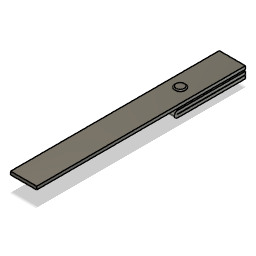
light v1 (Autodesk Fusion 360 design; units mm, degrees)
Autodesk Fusion 360 part; units mm, degrees
sketch "Esquisse1" plane through (0, 0, 0) normal (0, 1, 0) x (1, 0, 0)
  line L0 (25, 200) -> (-25, 200)
  line L1 (-25, 200) -> (-25, -200)
  line L2 (-25, -200) -> (25, -200)
  line L3 (25, -200) -> (25, 200)
  line L4 (25, 200) -> (-25, -200) construction
  line L5 (-25, 200) -> (25, -200) construction
  circle A0 centre (0, 100) radius 6.5
  circle A1 centre (0, 100) radius 4
  dimension "d1" = 50
  dimension "d2" = 400
  dimension "d3" = 13
  dimension "d4" = 8
  constraint horizontal L0
  constraint perpendicular L0 L1
  constraint parallel L0 L2
  constraint parallel L1 L3
  constraint coincident L4 origin
  constraint coincident L5 origin
  constraint concentric A0 A1
  measures "d1" distance of L1.end L2.end
  measures "d2" distance of L0.end L1.end
  measures "d3" diameter of A0
  measures "d4" diameter of A1
extrude "Extrusion1" add sketch "Esquisse1" against normal blind 6 contours L0 L1 L2 L3 makes body 1
extrude "Extrusion2" add sketch "Esquisse1" against normal blind 7 contours A0 bodies 1
fillet "Congé1" radius 3 1 edges at (-6.0601, -7, -102.3505) on bodies 1
extrude "Extrusion3" add 1 faces at (0.1619, -6, 102.1606) along direction (0, -1, 0) blind 9 and the other way blind -3 on bodies 1 bodies 1 makes body 2
extrude "Extrusion4" add sketch "Esquisse1" along normal blind -15 and the other way blind 8 contours A0 bodies 2
fillet "Congé2" radius 3 1 edges at (-6.0601, -8, -102.3505) on bodies 2
extrude "Extrusion5" add 1 faces at (0, -15, 101.3333) along direction (0, -1, 0) blind 6.5 and the other way blind -0.5 separate body on bodies 2 makes body 3
extrude "Extrusion6" add sketch "Esquisse1" along normal blind -22.5 and the other way blind 15.5 contours A0 bodies 3
fillet "Congé3" radius 3 1 edges at (-6.0601, -22.5, -102.3505) on bodies 3
extrude "Extrusion7" add sketch "Esquisse1" along normal blind 1 contours A0 bodies 1
fillet "Congé4" radius 3 1 edges at (-6.0601, 1, -97.6495) on bodies 1
extrude "Extrusion8" cut 2 faces at (-8.3333, -17.5, 200) (-8.3333, -11, 200) along direction (0, 0, -1) blind 270 on bodies 2 3 bodies 2 3
extrude "Extrusion9" add 1 faces at (-0.0996, -15, -167.9963) along direction (0, -1, 0) blind 0.25 separate body on bodies 2 makes body 4
revolve "Révolution1" add 1 faces at (-8.3333, -11, -70) angle 180 about axis through (25, -15.25, -70) along (1, 0, 0) on bodies 2 bodies 2 3 4
extrude "Extrusion10" cut 1 faces at (-0.0996, -15.25, -167.9963) along direction (0, 1, 0) blind 0.25 on bodies 2 bodies 2
sketch "Esquisse2" plane through (0, 0, 0) normal (0, -1, 0) x (1, 0, 0)
  line L0 (25, -70) -> (-25, -70)
  line L1 (-25, -70) -> (-25, -200)
  line L2 (-25, -200) -> (25, -200)
  line L3 (25, -200) -> (25, -70)
  circle A0 centre (0, -100) radius 6.5
  circle A1 centre (0, -100) radius 10
  circle A2 centre (0, -100) radius 3.5
  circle A3 centre (0, -100) radius 6.5
  line L4 (25, 200) -> (25, -200)
  line L5 (25, -200) -> (-25, -200)
  line L6 (-25, -200) -> (-25, 200)
  line L7 (-25, 200) -> (25, 200)
  dimension "d42" = 7
  constraint concentric A0 A1
  constraint concentric A1 A2
  measures "d42" diameter of A2
extrude "Extrusion11" add sketch "Esquisse2" along normal blind -1 and the other way blind 4 separate body contours A0 A3 | A1 | A2 makes body 5
fillet "Congé5" radius 2 1 edges at (-9.3233, 4, -96.3838) on bodies 5
fillet "Congé6" radius 1 1 edges at (-9.3233, 1, -96.3838) on bodies 5
extrude "Extrusion12" add sketch "Esquisse2" along normal blind 22.5 and the other way blind 1 contours A2 bodies 5
extrude "Extrusion13" add 1 faces at (1.7216, -22.5, -100.6592) along direction (0, -1, 0) blind 12 on bodies 5 bodies 5
ref_plane "Plan de construction1" through (0, 0, -100) normal (0, 0, 1) x (1, 0, 0)
sketch "Esquisse3" plane through (0, 0, -100) normal (0, 0, 1) x (1, 0, 0)
  line L0 (0, -32.5) -> (0, -22.5)
  line L1 (0, -22.5) -> (0, -22.7)
  circle A0 centre (0, -25.5) radius 1.7
  line L2 (0, -34.5) -> (-1.5, -34.5)
  line L3 (-1.5, -34.5) -> (-1.5, -32.5)
  circle A1 centre (-1.5, -32.5) radius 2
  circle A2 centre (1.5, -32.5) radius 2
  line L4 (3.5, -34.5) -> (3.5, -31.3)
  line L5 (-3.5, -34.5) -> (3.5, -34.5)
  line L6 (3.5, -34.5) -> (-3.5, -34.5)
  line L7 (-3.5, -34.5) -> (-3.5, -31.3)
  dimension "d60" = 3.4
  dimension "d65" = 1.5
  dimension "d66" = 2
  dimension "d67" = 4
  constraint vertical L0
  constraint coincident L0 L1.end
  constraint horizontal L2
  constraint perpendicular L2 L3
  constraint coincident L3.end A1.centre
  constraint symmetric L0 A1 A2
  constraint vertical L4
  constraint tangent A2 L4
  constraint coincident L4.start L5
  constraint coincident L4.start L5.end
  constraint coincident L5.start L6.end
  constraint perpendicular L6 L7
  constraint coincident L0 A0.centre
  measures "d60" diameter of A0
  measures "d65" distance of L2.start L2.end
  measures "d66" distance of L2.end L3.end
  measures "d67" diameter of A1
extrude "Extrusion14" cut sketch "Esquisse3" along normal blind 5 and the other way blind 5 contours L0 A0 | L0 A0 bodies 5
thread "Filetage2" "ISO Metric profile 7.0 M7x1 6g" major diameter 6.884 minor diameter 5.744 pitch 1 angle 60 modelled right hand crest width 0.1446 on face at (-2.0275, -19.6639, -102.8529) crest through (3.442, 1.25, -100) on bodies 5
revolve "Révolution2" cut sketch "Esquisse3" angle 360 about axis through (0, -32.5, -100) along (0, 1, 0) contours A1 L5 L6 L7 | A2 L4 L5 L6 bodies 5
sketch "Esquisse5" plane through (0, -34.5, 0) normal (0, -1, 0) x (1, 0, 0)
  circle A0 centre (0, -100) radius 1.5
  circle A1 centre (0, -100) radius 10
  circle A2 centre (0, -100) radius 3.5
  circle A3 centre (0, -100) radius 5.5
  circle A4 centre (0, -100) radius 9
  circle A5 centre (0, -100) radius 8.9
  line L0 (0, -108.9) -> (7.7076, -104.45)
  line L1 (7.7076, -104.45) -> (7.7076, -95.55)
  line L2 (7.7076, -95.55) -> (0, -91.1)
  line L3 (0, -91.1) -> (-7.7076, -95.55)
  line L4 (-7.7076, -95.55) -> (-7.7076, -104.45)
  line L5 (-7.7076, -104.45) -> (0, -108.9)
  line L6 (0, -109) -> (7.7942, -104.5)
  line L7 (7.7942, -104.5) -> (7.7942, -95.5)
  line L8 (7.7942, -95.5) -> (0, -91)
  line L9 (0, -91) -> (-7.7942, -95.5)
  line L10 (-7.7942, -95.5) -> (-7.7942, -104.5)
  line L11 (-7.7942, -104.5) -> (0, -109)
  point P0 (0, -100)
  point P1 (0, -100)
  dimension "d69" = 20
  dimension "d70" = 7
  dimension "d71" = 11
  dimension "d94" = -1
  dimension "d95" = -1.1
  constraint concentric A0 A1
  constraint concentric A1 A2
  constraint concentric A1 A3
  constraint coincident P1 P0
  constraint coincident A5 L0.start
  constraint coincident A4 L6.start
  measures "d69" diameter of A1
  measures "d70" diameter of A2
  measures "d71" diameter of A3
extrude "Extrusion16" add sketch "Esquisse5" against normal blind 7 separate body contours A2 | A3 | L0 L1 L2 L3 L4 L5 makes body 6
extrude "Extrusion19" add sketch "Esquisse5" against normal blind 7 separate body contours A1 | A4 A5 L7 | A4 A5 L8 | A4 A5 L6 | A4 A5 L9 | A5 L7 | A5 L8 | A4 A5 L11 | A5 L6 | A4 A5 L10 | A5 L9 | A5 L11 | A5 L10 makes body 7
extrude "Extrusion18" add sketch "Esquisse5" along normal blind 1 contours A0 | A1 | A2 | A3 | A4 A5 L7 | A4 A5 L8 | A5 L7 L8 | A4 A5 L6 | A5 L6 L7 | A4 A5 L9 | A5 L8 L9 | A5 L1 L7 | A5 L7 | A5 L8 | A5 L2 L8 | A5 L6 L11 | A4 A5 L11 | A5 L0 L6 | A5 L6 | A4 A5 L10 | A5 L9 L10 | A5 L9 | A5 L3 L9 | L0 L1 L2 L3 L4 L5 | A5 L10 L11 | A5 L5 L11 | A5 L11 | A5 L10 | A5 L4 L10 bodies 7
chamfer "Chanfrein1" distance 0.5 angle 45 1 edges at (-9.3233, -35.5, -103.6162) on bodies 7
thread "Filetage4" "ISO Metric profile 7.0 M7x1 6H" major diameter 7.1472 minor diameter 6.0355 pitch 1 angle 60 modelled right hand crest width 0.2748 on face at (-1.3822, -29.8333, -99.4173) crest through (3.0178, -34.25, -100) on bodies 6
sketch "Esquisse8" plane through (0, -35.5, 0) normal (0, -1, 0) x (1, 0, 0)
  circle A0 centre (0, -100) radius 9.5
  line L0 (2.1529, -103.726) -> (-0.1022, -103.7247)
  line L1 (-0.127, -102.8894) -> (4.5454, -102.9017)
  line L2 (-0.111, -93.9025) -> (0.5539, -93.9025)
  line L3 (-2.3574, -103.7233) -> (-2.561, -103.942)
  line L4 (-5.3603, -104.1349) -> (-5.7439, -103.5844)
  line L5 (0.5539, -93.9025) -> (1.0031, -94.5435)
  line L6 (2.3659, -99.2001) -> (1.1685, -97.2165)
  line L7 (1.8541, -95.7782) -> (2.2558, -96.3718)
  line L8 (1.1685, -97.2165) -> (-0.0289, -95.2329)
  line L9 (-2.561, -103.942) -> (-2.7647, -104.1607)
  line L10 (-4.7994, -102.877) -> (-0.127, -102.8894)
  line L11 (-2.4474, -98.9824) -> (-3.0749, -100.0226)
  line L12 (-3.5593, -99.1034) -> (-2.7615, -97.8938)
  line L13 (5.1426, -104.1591) -> (3.8384, -104.1591)
  line L14 (2.8468, -99.9984) -> (2.3659, -99.2001)
  line L15 (3.1814, -98.8624) -> (4.1069, -100.2645)
  line L16 (-0.1022, -103.7247) -> (-2.3574, -103.7233)
  line L17 (1.0031, -94.5435) -> (1.4523, -95.1845)
  line L18 (5.9218, -103.0086) -> (5.5322, -103.5838)
  line L19 (-4.3571, -100.3129) -> (-3.5593, -99.1034)
  line L20 (2.2558, -96.3718) -> (2.2558, -96.916)
  line L21 (-0.0521, -95.1941) -> (-0.0753, -95.1552)
  line L22 (-0.0753, -95.1552) -> (-0.117, -95.1699)
  line L23 (4.3334, -102.4614) -> (4.0822, -102.0604)
  line L24 (1.4523, -95.1845) -> (1.8541, -95.7782)
  line L25 (-2.7647, -104.1607) -> (-4.0625, -104.1478)
  line L26 (2.2558, -96.916) -> (2.2558, -97.4602)
  line L27 (-4.0625, -104.1478) -> (-5.3603, -104.1349)
  line L28 (5.0143, -101.6365) -> (5.9218, -103.0086)
  line L29 (2.2558, -97.4602) -> (3.1814, -98.8624)
  line L30 (-0.0289, -95.2329) -> (-0.0521, -95.1941)
  line L31 (3.8384, -104.1591) -> (2.5341, -104.1591)
  line L32 (-2.437, -96.8474) -> (-2.437, -96.2947)
  line L33 (4.1069, -100.2645) -> (5.0143, -101.6365)
  line L34 (3.5941, -101.2321) -> (3.3276, -100.7967)
  line L35 (-2.437, -97.4) -> (-2.437, -96.8474)
  line L36 (4.5847, -102.8623) -> (4.3334, -102.4614)
  line L37 (5.5322, -103.5838) -> (5.1426, -104.1591)
  line L38 (-3.0749, -100.0226) -> (-3.9372, -101.4498)
  line L39 (-6.1275, -103.034) -> (-6.0391, -102.8829)
  line L40 (4.0822, -102.0604) -> (3.9714, -101.864)
  line L41 (4.565, -102.882) -> (4.5847, -102.8623)
  line L42 (-0.9892, -96.5634) -> (-1.8198, -97.9422)
  line L43 (-0.117, -95.1699) -> (-0.1587, -95.1845)
  line L44 (3.3276, -100.7967) -> (2.8468, -99.9984)
  line L45 (-5.9508, -102.7319) -> (-5.1539, -101.5224)
  line L46 (-2.7615, -97.8938) -> (-2.5993, -97.6469)
  line L47 (2.5341, -104.1591) -> (2.3435, -103.9425)
  line L48 (2.3435, -103.9425) -> (2.1529, -103.726)
  line L49 (-0.7759, -93.9025) -> (-0.111, -93.9025)
  line L50 (4.5454, -102.9017) -> (4.565, -102.882)
  line L51 (-1.8198, -97.9422) -> (-2.4474, -98.9824)
  line L52 (-2.5993, -97.6469) -> (-2.437, -97.4)
  line L53 (3.9714, -101.864) -> (3.8606, -101.6675)
  line L54 (-1.6065, -95.0986) -> (-0.7759, -93.9025)
  line L55 (-0.1587, -95.1845) -> (-0.9892, -96.5634)
  line L56 (3.8606, -101.6675) -> (3.5941, -101.2321)
  line L57 (-3.9372, -101.4498) -> (-4.7994, -102.877)
  line L58 (-5.1539, -101.5224) -> (-4.3571, -100.3129)
  line L59 (-2.437, -96.2947) -> (-1.6065, -95.0986)
  line L60 (-6.0391, -102.8829) -> (-5.9508, -102.7319)
  line L61 (-5.7439, -103.5844) -> (-6.1275, -103.034)
  line L62 (0.026, -99.3269) -> (0.1067, -99.0458)
  line L63 (0.1067, -99.0458) -> (0.1873, -98.7647)
  line L64 (1.3787, -99.2969) -> (1.3509, -99.4178)
  line L65 (0.2142, -98.734) -> (0.4972, -98.6664)
  line L66 (0.2768, -100.3854) -> (-0.1004, -100.3847)
  line L67 (0.8286, -98.6012) -> (0.877, -98.6036)
  line L68 (0.2768, -100.3854) -> (-0.1004, -100.3847)
  line L69 (1.0463, -98.7229) -> (1.2157, -98.8422)
  line L70 (1.2157, -98.8422) -> (1.2972, -99.0696)
  line L71 (1.2157, -98.8422) -> (1.2972, -99.0696)
  line L72 (0.8286, -98.6012) -> (0.877, -98.6036)
  line L73 (1.3787, -99.2969) -> (1.3509, -99.4178)
  line L74 (0.2008, -98.7493) -> (0.2142, -98.734)
  line L75 (0.4658, -102.1164) -> (0.3706, -102.2306)
  line L76 (0.4972, -98.6664) -> (0.7803, -98.5988)
  line L77 (0.2739, -102.1876) -> (0.2723, -102.0304)
  line L78 (-0.358, -100.7048) -> (-0.3188, -100.9926)
  line L79 (0.2755, -102.3448) -> (0.2739, -102.1876)
  line L80 (0.2142, -98.734) -> (0.4972, -98.6664)
  line L81 (-1.3171, -100.9376) -> (-1.5364, -101.1154)
  line L82 (1.6586, -100.4178) -> (1.6881, -100.8009)
  line L83 (1.3509, -99.4178) -> (1.323, -99.5388)
  line L84 (-1.4452, -99.7767) -> (-1.5302, -99.6094)
  line L85 (1.2972, -99.0696) -> (1.3787, -99.2969)
  line L86 (1.0887, -100.9285) -> (0.893, -100.7459)
  line L87 (0.0787, -101.0119) -> (0.0787, -100.6912)
  line L88 (-0.3642, -99.0351) -> (-0.2755, -99.2969)
  line L89 (0.1067, -99.0458) -> (0.1873, -98.7647)
  line L90 (0.3706, -102.2306) -> (0.2755, -102.3448)
  line L91 (0.026, -99.3269) -> (0.1067, -99.0458)
  line L92 (-1.4452, -99.7767) -> (-1.5302, -99.6094)
  line L93 (-0.1248, -99.3119) -> (0.026, -99.3269)
  line L94 (1.2972, -99.0696) -> (1.3787, -99.2969)
  line L95 (1.3509, -99.4178) -> (1.323, -99.5388)
  line L96 (-1.7306, -101.0869) -> (-1.8219, -100.9302)
  line L97 (1.0463, -98.7229) -> (1.2157, -98.8422)
  line L98 (-0.6265, -100.6273) -> (-0.5521, -100.6281)
  line L99 (-0.4528, -98.7734) -> (-0.3642, -99.0351)
  line L100 (-0.8406, -99.9035) -> (-0.9494, -99.8781)
  line L101 (0.877, -98.6036) -> (1.0463, -98.7229)
  line L102 (-1.0851, -98.5958) -> (-0.7885, -98.665)
  line L103 (-1.4653, -98.8358) -> (-1.2752, -98.7158)
  line L104 (-0.8406, -99.9035) -> (-0.9494, -99.8781)
  line L105 (0.7803, -98.5988) -> (0.8286, -98.6012)
  line L106 (-0.492, -98.7342) -> (-0.4724, -98.7538)
  line L107 (-0.3338, -101.5494) -> (-0.3879, -101.8183)
  line L108 (-1.5662, -101.2079) -> (-1.5662, -101.3869)
  line L109 (-0.3642, -99.0351) -> (-0.2755, -99.2969)
  line L110 (0.877, -98.6036) -> (1.0463, -98.7229)
  line L111 (0.1873, -98.7647) -> (0.2008, -98.7493)
  line L112 (-0.2755, -99.2969) -> (-0.1248, -99.3119)
  line L113 (0.1873, -98.7647) -> (0.2008, -98.7493)
  line L114 (-1.5914, -99.2344) -> (-1.5675, -99.0269)
  line L115 (0.7803, -98.5988) -> (0.8286, -98.6012)
  line L116 (-0.2755, -99.2969) -> (-0.1248, -99.3119)
  line L117 (0.4972, -98.6664) -> (0.7803, -98.5988)
  line L118 (0.2008, -98.7493) -> (0.2142, -98.734)
  line L119 (0.355, -100.579) -> (0.6039, -100.8421)
  line L120 (-0.9697, -101.0386) -> (-0.7981, -100.8329)
  line L121 (-0.4724, -98.7538) -> (-0.4528, -98.7734)
  line L122 (-1.0851, -98.5958) -> (-0.7885, -98.665)
  line L123 (-0.4724, -98.7538) -> (-0.4528, -98.7734)
  line L124 (-1.6152, -99.442) -> (-1.5914, -99.2344)
  line L125 (-0.4776, -100.3839) -> (-0.5309, -100.3484)
  line L126 (-1.7218, -101.2079) -> (-1.644, -101.2079)
  line L127 (0.5142, -99.9919) -> (0.4416, -100.0846)
  line L128 (0.3252, -100.579) -> (0.3401, -100.579)
  line L129 (-1.8444, -100.0393) -> (-1.7446, -99.9463)
  line L130 (1.2845, -101.1111) -> (1.0887, -100.9285)
  line L131 (-1.052, -101.4228) -> (-1.0691, -101.2321)
  line L132 (0.369, -102.0304) -> (0.4658, -102.0304)
  line L133 (0.5867, -99.8992) -> (0.5142, -99.9919)
  line L134 (-1.6335, -101.1012) -> (-1.7306, -101.0869)
  line L135 (0.4416, -100.0846) -> (0.3592, -100.235)
  line L136 (0.893, -100.7459) -> (0.8729, -100.481)
  line L137 (0.202, -100.6351) -> (0.3252, -100.579)
  line L138 (-1.6112, -101.5199) -> (-1.6561, -101.474)
  line L139 (1.4156, -101.2065) -> (1.3378, -101.2065)
  line L140 (1.3378, -101.2065) -> (1.3378, -101.3855)
  line L141 (1.6881, -100.8009) -> (1.6079, -100.956)
  line L142 (-1.0879, -100.4842) -> (-1.0978, -100.7597)
  line L143 (0.8729, -100.481) -> (0.8528, -100.2161)
  line L144 (0.7242, -101.7216) -> (0.5957, -101.8902)
  line L145 (-1.3318, -100.031) -> (-1.0779, -100.2088)
  line L146 (-1.0582, -99.8528) -> (-1.2517, -99.8148)
  line L147 (1.6079, -100.956) -> (1.5277, -101.1111)
  line L148 (0.8528, -101.1053) -> (0.8528, -101.3292)
  line L149 (0.0787, -100.6912) -> (0.202, -100.6351)
  line L150 (-1.0978, -100.7597) -> (-1.3171, -100.9376)
  line L151 (-0.1004, -100.3847) -> (-0.4776, -100.3839)
  line L152 (1.1985, -99.7865) -> (0.8926, -99.8429)
  line L153 (-0.592, -101.9336) -> (-0.7247, -101.9336)
  line L154 (0.3592, -100.235) -> (0.2768, -100.3854)
  line L155 (1.5433, -99.9697) -> (1.629, -100.0348)
  line L156 (1.4277, -101.4725) -> (1.4606, -101.3395)
  line L157 (-0.7123, -100.1082) -> (-0.8406, -99.9035)
  line L158 (-1.0779, -100.2088) -> (-1.0879, -100.4842)
  line L159 (0.8528, -101.3292) -> (0.8528, -101.553)
  line L160 (-1.689, -101.3409) -> (-1.7218, -101.2079)
  line L161 (-1.5662, -101.5659) -> (-1.6112, -101.5199)
  line L162 (1.3378, -101.5645) -> (1.3828, -101.5185)
  line L163 (0.5142, -99.9919) -> (0.4416, -100.0846)
  line L164 (1.0942, -100.0589) -> (1.3356, -99.9016)
  line L165 (1.629, -100.0348) -> (1.6586, -100.4178)
  line L166 (-0.4534, -101.982) -> (-0.4534, -102.1513)
  line L167 (-0.5948, -102.027) -> (-0.526, -101.9835)
  line L168 (-1.6447, -99.8532) -> (-1.6152, -99.8532)
  line L169 (-0.4235, -101.8759) -> (-0.4592, -101.9336)
  line L170 (-1.9132, -100.7734) -> (-1.8788, -100.4064)
  line L171 (-0.5816, -102.1956) -> (-0.6635, -102.0705)
  line L172 (-0.4592, -101.9336) -> (-0.592, -101.9336)
  line L173 (-1.0582, -99.8528) -> (-1.2517, -99.8148)
  line L174 (0.2642, -101.861) -> (0.1715, -101.5968)
  line L175 (1.1985, -99.7865) -> (0.8926, -99.8429)
  line L176 (-0.7247, -101.9336) -> (-0.8798, -101.7736)
  line L177 (0.1715, -101.5968) -> (0.0787, -101.3326)
  line L178 (-1.6152, -99.8532) -> (-1.5858, -99.8532)
  line L179 (1.4606, -101.3395) -> (1.4934, -101.2065)
  line L180 (-0.4897, -101.9827) -> (-0.4534, -101.982)
  line L181 (0.4658, -102.0734) -> (0.4658, -102.1164)
  line L182 (-0.9494, -99.8781) -> (-1.0582, -99.8528)
  line L183 (0.5957, -101.8902) -> (0.4299, -101.8756)
  line L184 (0.2723, -102.0304) -> (0.369, -102.0304)
  line L185 (-0.3879, -101.8183) -> (-0.4235, -101.8759)
  line L186 (-0.6635, -102.0705) -> (-0.5948, -102.027)
  line L187 (1.3966, -99.9032) -> (1.4576, -99.9047)
  line L188 (-1.8219, -100.9302) -> (-1.9132, -100.7734)
  line L189 (-0.4534, -102.1513) -> (-0.4534, -102.3206)
  line L190 (-0.4765, -102.3206) -> (-0.4996, -102.3206)
  line L191 (-0.4534, -102.3206) -> (-0.4765, -102.3206)
  line L192 (-0.526, -101.9835) -> (-0.4897, -101.9827)
  line L193 (-0.4996, -102.3206) -> (-0.5816, -102.1956)
  line L194 (1.5277, -101.1111) -> (1.4061, -101.1111)
  line L195 (0.4658, -102.0304) -> (0.4658, -102.0734)
  line L196 (-1.2517, -99.8148) -> (-1.4452, -99.7767)
  line L197 (1.3378, -101.3855) -> (1.3378, -101.5645)
  line L198 (0.4416, -100.0846) -> (0.3592, -100.235)
  line L199 (-0.5309, -100.3484) -> (-0.5841, -100.3129)
  line L200 (-0.7981, -100.8329) -> (-0.6265, -100.6273)
  line L201 (0.3592, -100.235) -> (0.2768, -100.3854)
  line L202 (0.8528, -100.2161) -> (1.0942, -100.0589)
  line L203 (-1.5302, -99.6094) -> (-1.6152, -99.442)
  line L204 (-0.5841, -100.3129) -> (-0.7123, -100.1082)
  line L205 (-0.9494, -99.8781) -> (-1.0582, -99.8528)
  line L206 (-1.2752, -98.7158) -> (-1.0851, -98.5958)
  line L207 (1.4576, -99.9047) -> (1.5433, -99.9697)
  line L208 (-1.5675, -99.0269) -> (-1.5164, -98.9314)
  line L209 (1.4061, -101.1111) -> (1.2845, -101.1111)
  line L210 (-1.2517, -99.8148) -> (-1.4452, -99.7767)
  line L211 (-0.4776, -100.3839) -> (-0.5309, -100.3484)
  line L212 (-1.5164, -98.9314) -> (-1.4653, -98.8358)
  line L213 (0.5867, -99.8992) -> (0.5142, -99.9919)
  line L214 (0.8528, -101.553) -> (0.7242, -101.7216)
  line L215 (0.3401, -100.579) -> (0.355, -100.579)
  line L216 (1.2608, -99.6626) -> (1.1985, -99.7865)
  line L217 (-1.6561, -101.474) -> (-1.689, -101.3409)
  line L218 (-1.5302, -99.6094) -> (-1.6152, -99.442)
  line L219 (-1.5364, -101.1154) -> (-1.6335, -101.1012)
  line L220 (-0.3188, -100.9926) -> (-0.2797, -101.2805)
  line L221 (-1.8788, -100.4064) -> (-1.8444, -100.0393)
  line L222 (1.3828, -101.5185) -> (1.4277, -101.4725)
  line L223 (1.323, -99.5388) -> (1.2608, -99.6626)
  line L224 (-0.1004, -100.3847) -> (-0.4776, -100.3839)
  line L225 (-1.5675, -99.0269) -> (-1.5164, -98.9314)
  line L226 (-1.0691, -101.2321) -> (-1.0194, -101.1353)
  line L227 (-0.7123, -100.1082) -> (-0.8406, -99.9035)
  line L228 (-0.4528, -98.7734) -> (-0.3642, -99.0351)
  line L229 (-1.5914, -99.2344) -> (-1.5675, -99.0269)
  line L230 (-0.1248, -99.3119) -> (0.026, -99.3269)
  line L231 (0.6039, -100.8421) -> (0.8528, -101.1053)
  line L232 (1.323, -99.5388) -> (1.2608, -99.6626)
  line L233 (-1.5662, -101.3869) -> (-1.5662, -101.5659)
  line L234 (-1.4653, -98.8358) -> (-1.2752, -98.7158)
  line L235 (-1.644, -101.2079) -> (-1.5662, -101.2079)
  line L236 (-0.4178, -100.6668) -> (-0.358, -100.7048)
  line L237 (-0.7885, -98.665) -> (-0.492, -98.7342)
  line L238 (-1.5164, -98.9314) -> (-1.4653, -98.8358)
  line L239 (0.0787, -101.3326) -> (0.0787, -101.0119)
  line L240 (-0.492, -98.7342) -> (-0.4724, -98.7538)
  line L241 (-1.7446, -99.9463) -> (-1.6447, -99.8532)
  line L242 (1.2608, -99.6626) -> (1.1985, -99.7865)
  line L243 (-0.7885, -98.665) -> (-0.492, -98.7342)
  line L244 (-0.5521, -100.6281) -> (-0.4776, -100.6288)
  line L245 (-0.4776, -100.6288) -> (-0.4178, -100.6668)
  line L246 (1.3356, -99.9016) -> (1.3966, -99.9032)
  line L247 (-1.0349, -101.6136) -> (-1.052, -101.4228)
  line L248 (0.8926, -99.8429) -> (0.5867, -99.8992)
  line L249 (-0.5841, -100.3129) -> (-0.7123, -100.1082)
  line L250 (-0.2797, -101.2805) -> (-0.3338, -101.5494)
  line L251 (0.4299, -101.8756) -> (0.2642, -101.861)
  line L252 (-1.0194, -101.1353) -> (-0.9697, -101.0386)
  line L253 (1.4934, -101.2065) -> (1.4156, -101.2065)
  line L254 (-0.5309, -100.3484) -> (-0.5841, -100.3129)
  line L255 (-1.6152, -99.442) -> (-1.5914, -99.2344)
  line L256 (-1.5858, -99.8532) -> (-1.3318, -100.031)
  line L257 (-0.8798, -101.7736) -> (-1.0349, -101.6136)
  line L258 (0.8926, -99.8429) -> (0.5867, -99.8992)
  line L259 (-1.2752, -98.7158) -> (-1.0851, -98.5958)
  dimension "d114" = 0
emboss "Gravure en relief2" depth -0.4 profiles "Esquisse8" section 1 contours L0 L2 L3 L4 L5 L7 L9 L12 L13 L15 L16 L17 L18 L19 L20 L24 L25 L26 L27 L28 L29 L31 L32 L33 L35 L37 L39 L45 L46 L47 L48 L49 L52 L54 L58 L59 L60 L61 | L62 L63 L64 L65 L66 L67 L68 L69 L70 L71 L72 L73 L74 L76 L80 L83 L84 L85 L88 L89 L91 L92 L93 L94 L95 L97 L99 L100 L101 L102 L103 L104 L105 L106 L109 L110 L111 L112 L113 L114 L115 L116 L117 L118 L121 L122 L123 L124 L125 L127 L133 L135 L146 L151 L152 L154 L157 L163 L173 L175 L182 L196 L198 L199 L201 L203 L204 L205 L206 L208 L210 L211 L212 L213 L216 L218 L223 L224 L225 L227 L228 L229 L230 L232 L234 L237 L238 L240 L242 L243 L248 L249 L254 L255 L258 L259 | L75 L77 L79 L90 L132 L181 L184 L195 | L78 L98 L107 L120 L131 L153 L169 L172 L176 L185 L200 L220 L226 L236 L244 L245 L247 L250 L252 L257 | L81 L96 L129 L134 L142 L145 L150 L158 L168 L170 L178 L188 L219 L221 L241 L256 | L82 L86 L130 L136 L141 L143 L147 L155 L164 L165 L187 L194 L202 L207 L209 L246 | L87 L119 L128 L137 L144 L148 L149 L159 L174 L177 L183 L214 L215 L231 L239 L251 | L108 L126 L138 L160 L161 L217 L233 L235 | L139 L140 L156 L162 L179 L197 L222 L253 | L166 L167 L171 L180 L186 L189 L190 L191 L192 L193 onto face at (-0.0584, -35.5, -92.9045) on bodies 7 bodies 7
sketch "Esquisse9" plane through (0, 0, 0) normal (0, 0, 1) x (1, 0, 0)
  spline S0 degree 3 poles (5.4127, -28.6266) (5.517, -28.731) (5.5206, -28.7549) (5.5192, -29.3414) knots 0 0 0 0 1 1 1 1
  spline S1 degree 3 poles (5.5192, -29.3414) (5.5173, -30.1912) (5.5184, -30.1902) (4.5558, -30.1902) knots 0 0 0 0 1 1 1 1
  line L0 (4.5558, -30.1902) -> (3.8931, -30.1902)
  line L1 (3.8931, -30.1902) -> (3.8931, -30.0142)
  line L2 (3.8931, -30.0142) -> (3.8931, -29.8383)
  line L3 (3.8931, -29.8383) -> (4.5309, -29.8383)
  line L4 (4.5309, -29.8383) -> (5.1687, -29.8383)
  line L5 (5.1687, -29.8383) -> (5.1687, -29.3544)
  line L6 (5.1687, -29.3544) -> (5.1687, -28.8705)
  line L7 (5.1687, -28.8705) -> (4.5309, -28.8705)
  line L8 (4.5309, -28.8705) -> (3.8931, -28.8705)
  line L9 (3.8931, -28.8705) -> (3.8931, -28.6946)
  line L10 (3.8931, -28.6946) -> (3.8931, -28.5186)
  line L11 (3.8931, -28.5186) -> (4.5989, -28.5186)
  spline S2 degree 3 poles (4.5989, -28.5186) (5.2896, -28.5186) (5.307, -28.521) (5.4127, -28.6266) knots 0 0 0 0 1 1 1 1
  spline S3 degree 3 poles (3.4312, -28.5712) (3.4796, -28.5986) (3.5337, -28.6426) (3.5515, -28.6688) knots 0 0 0 0 1 1 1 1
  spline S4 degree 3 poles (3.5515, -28.6688) (3.5693, -28.6951) (3.5841, -29.0055) (3.5845, -29.3586) knots 0 0 0 0 1 1 1 1
  spline S5 degree 3 poles (3.5845, -29.3586) (3.5853, -30.1868) (3.6064, -30.1624) (2.8729, -30.183) knots 0 0 0 0 1 1 1 1
  spline S6 degree 3 poles (2.8729, -30.183) (2.283, -30.1995) (2.1696, -30.1823) (2.0445, -30.0571) knots 0 0 0 0 1 1 1 1
  spline S7 degree 3 poles (2.0445, -30.0571) (1.9662, -29.9789) (1.9576, -29.9089) (1.9576, -29.3524) knots 0 0 0 0 1 1 1 1
  spline S8 degree 3 poles (1.9576, -29.3524) (1.9576, -28.7551) (1.9612, -28.731) (2.0656, -28.6266) knots 0 0 0 0 1 1 1 1
  spline S9 degree 3 poles (2.0656, -28.6266) (2.1695, -28.5226) (2.1952, -28.5187) (2.7584, -28.52) knots 0 0 0 0 1 1 1 1
  spline S10 degree 3 poles (2.7584, -28.52) (3.1108, -28.5208) (3.3782, -28.5411) (3.4312, -28.5712) knots 0 0 0 0 1 1 1 1
  line L12 (2.3095, -29.3544) -> (2.3095, -29.8383)
  line L13 (2.3095, -29.8383) -> (2.7934, -29.8383)
  line L14 (2.7934, -29.8383) -> (3.2772, -29.8383)
  line L15 (3.2772, -29.8383) -> (3.2772, -29.3544)
  line L16 (3.2772, -29.3544) -> (3.2772, -28.8705)
  line L17 (3.2772, -28.8705) -> (2.7934, -28.8705)
  line L18 (2.7934, -28.8705) -> (2.3095, -28.8705)
  line L19 (2.3095, -28.8705) -> (2.3095, -29.3544)
  line L20 (1.6497, -29.3544) -> (1.6497, -30.1902)
  line L21 (1.6497, -30.1902) -> (1.5047, -30.1902)
  spline S11 degree 3 poles (1.5047, -30.1902) (1.3408, -30.1902) (1.2589, -30.1146) (0.7219, -29.4677) knots 0 0 0 0 1 1 1 1
  line L22 (0.7219, -29.4677) -> (0.396, -29.0751)
  line L23 (0.396, -29.0751) -> (0.374, -29.6217)
  line L24 (0.374, -29.6217) -> (0.352, -30.1682)
  line L25 (0.352, -30.1682) -> (0.1871, -30.1818)
  line L26 (0.1871, -30.1818) -> (0.0221, -30.1955)
  line L27 (0.0221, -30.1955) -> (0.0221, -29.3571)
  line L28 (0.0221, -29.3571) -> (0.0221, -28.5186)
  line L29 (0.0221, -28.5186) -> (0.1947, -28.5186)
  spline S12 degree 3 poles (0.1947, -28.5186) (0.3614, -28.5186) (0.3832, -28.5374) (0.8435, -29.0786) knots 0 0 0 0 1 1 1 1
  line L30 (0.8435, -29.0786) -> (1.3198, -29.6385)
  line L31 (1.3198, -29.6385) -> (1.3321, -29.0786)
  line L32 (1.3321, -29.0786) -> (1.3444, -28.5186)
  line L33 (1.3444, -28.5186) -> (1.497, -28.5186)
  line L34 (1.497, -28.5186) -> (1.6497, -28.5186)
  line L35 (1.6497, -28.5186) -> (1.6497, -29.3544)
  spline S13 degree 3 poles (-0.4017, -28.6098) (-0.2858, -28.701) (-0.2858, -28.7012) (-0.2858, -29.3508) knots 0 0 0 0 1 1 1 1
  spline S14 degree 3 poles (-0.2858, -29.3508) (-0.2858, -30.2109) (-0.2343, -30.1636) (-1.192, -30.1821) knots 0 0 0 0 1 1 1 1
  line L36 (-1.192, -30.1821) -> (-1.9133, -30.1961)
  line L37 (-1.9133, -30.1961) -> (-1.9133, -30.0172)
  line L38 (-1.9133, -30.0172) -> (-1.9133, -29.8383)
  line L39 (-1.9133, -29.8383) -> (-1.2535, -29.8383)
  line L40 (-1.2535, -29.8383) -> (-0.5937, -29.8383)
  line L41 (-0.5937, -29.8383) -> (-0.5937, -29.3544)
  line L42 (-0.5937, -29.3544) -> (-0.5937, -28.8705)
  line L43 (-0.5937, -28.8705) -> (-1.2535, -28.8705)
  line L44 (-1.2535, -28.8705) -> (-1.9133, -28.8705)
  line L45 (-1.9133, -28.8705) -> (-1.9133, -28.6946)
  line L46 (-1.9133, -28.6946) -> (-1.9133, -28.5186)
  line L47 (-1.9133, -28.5186) -> (-1.2155, -28.5186)
  spline S15 degree 3 poles (-1.2155, -28.5186) (-0.576, -28.5186) (-0.5079, -28.5263) (-0.4017, -28.6098) knots 0 0 0 0 1 1 1 1
  line L48 (-3.101, -29.1785) -> (-3.101, -29.8383)
  line L49 (-3.101, -29.8383) -> (-2.5732, -29.8383)
  line L50 (-2.5732, -29.8383) -> (-2.0453, -29.8383)
  line L51 (-2.0453, -29.8383) -> (-2.0453, -30.0142)
  line L52 (-2.0453, -30.0142) -> (-2.0453, -30.1902)
  line L53 (-2.0453, -30.1902) -> (-2.6112, -30.1902)
  spline S16 degree 3 poles (-2.6112, -30.1902) (-3.1171, -30.1902) (-3.1894, -30.1805) (-3.293, -30.099) knots 0 0 0 0 1 1 1 1
  line L54 (-3.293, -30.099) -> (-3.4089, -30.0078)
  line L55 (-3.4089, -30.0078) -> (-3.4089, -29.2632)
  line L56 (-3.4089, -29.2632) -> (-3.4089, -28.5186)
  line L57 (-3.4089, -28.5186) -> (-3.255, -28.5186)
  line L58 (-3.255, -28.5186) -> (-3.101, -28.5186)
  line L59 (-3.101, -28.5186) -> (-3.101, -29.1785)
  line L60 (-3.7269, -29.3434) -> (-3.7388, -30.1682)
  line L61 (-3.7388, -30.1682) -> (-4.4575, -30.1682)
  line L62 (-4.4575, -30.1682) -> (-5.1762, -30.1682)
  line L63 (-5.1762, -30.1682) -> (-5.2823, -30.0448)
  spline S17 degree 3 poles (-5.2823, -30.0448) (-5.4275, -29.8758) (-5.4369, -29.3839) (-5.2982, -29.2077) knots 0 0 0 0 1 1 1 1
  spline S18 degree 3 poles (-5.2982, -29.2077) (-5.2106, -29.0963) (-5.1923, -29.0927) (-4.6494, -29.0808) knots 0 0 0 0 1 1 1 1
  line L64 (-4.6494, -29.0808) -> (-4.0907, -29.0685)
  line L65 (-4.0907, -29.0685) -> (-4.0776, -28.7936)
  line L66 (-4.0776, -28.7936) -> (-4.0646, -28.5186)
  line L67 (-4.0646, -28.5186) -> (-3.8897, -28.5186)
  line L68 (-3.8897, -28.5186) -> (-3.7149, -28.5186)
  line L69 (-3.7149, -28.5186) -> (-3.7269, -29.3434)
  line L70 (-5.0279, -29.6293) -> (-5.0413, -29.8383)
  line L71 (-5.0413, -29.8383) -> (-4.555, -29.8383)
  line L72 (-4.555, -29.8383) -> (-4.0687, -29.8383)
  line L73 (-4.0687, -29.8383) -> (-4.0687, -29.6169)
  line L74 (-4.0687, -29.6169) -> (-4.0687, -29.3954)
  line L75 (-4.0687, -29.3954) -> (-4.5416, -29.4079)
  line L76 (-4.5416, -29.4079) -> (-5.0145, -29.4204)
  line L77 (-5.0145, -29.4204) -> (-5.0279, -29.6293)
  line L78 (5.6526, -32.3218) -> (5.6526, -34.0171)
  line L79 (5.6526, -34.0171) -> (4.1855, -34.0171)
  spline S19 degree 3 poles (4.1855, -34.0171) (2.7365, -34.0171) (2.7166, -34.0159) (2.573, -33.9181) knots 0 0 0 0 1 1 1 1
  spline S20 degree 3 poles (2.573, -33.9181) (2.2786, -33.7178) (2.2451, -33.6298) (2.2283, -33.0115) knots 0 0 0 0 1 1 1 1
  spline S21 degree 3 poles (2.2283, -33.0115) (2.2196, -32.6895) (2.2338, -32.3754) (2.2618, -32.2716) knots 0 0 0 0 1 1 1 1
  spline S22 degree 3 poles (2.2618, -32.2716) (2.3233, -32.0432) (2.6071, -31.7737) (2.7862, -31.7737) knots 0 0 0 0 1 1 1 1
  spline S23 degree 3 poles (2.7862, -31.7737) (2.8546, -31.7737) (2.9225, -31.7619) (2.9369, -31.7475) knots 0 0 0 0 1 1 1 1
  spline S24 degree 3 poles (2.9369, -31.7475) (2.9514, -31.733) (2.7963, -31.5243) (2.5924, -31.2837) knots 0 0 0 0 1 1 1 1
  spline S25 degree 3 poles (2.5924, -31.2837) (2.3465, -30.9937) (2.2215, -30.8099) (2.2215, -30.7382) knots 0 0 0 0 1 1 1 1
  spline S26 degree 3 poles (2.2215, -30.7382) (2.2215, -30.6315) (2.2268, -30.63) (2.6082, -30.63) knots 0 0 0 0 1 1 1 1
  line L80 (2.6082, -30.63) -> (2.995, -30.63)
  line L81 (2.995, -30.63) -> (3.4668, -31.2019)
  line L82 (3.4668, -31.2019) -> (3.9387, -31.7737)
  line L83 (3.9387, -31.7737) -> (4.4011, -31.7737)
  spline S27 degree 3 poles (4.4011, -31.7737) (4.7617, -31.7737) (4.8689, -31.7599) (4.8877, -31.7108) knots 0 0 0 0 1 1 1 1
  spline S28 degree 3 poles (4.8877, -31.7108) (4.901, -31.6762) (4.9152, -31.4238) (4.9193, -31.1499) knots 0 0 0 0 1 1 1 1
  line L84 (4.9193, -31.1499) -> (4.9268, -30.652)
  line L85 (4.9268, -30.652) -> (5.2897, -30.6393)
  line L86 (5.2897, -30.6393) -> (5.6526, -30.6265)
  line L87 (5.6526, -30.6265) -> (5.6526, -32.3218)
  line L88 (2.9693, -32.8954) -> (2.9693, -33.3133)
  line L89 (2.9693, -33.3133) -> (3.9371, -33.3133)
  spline S29 degree 3 poles (3.9371, -33.3133) (4.5511, -33.3133) (4.9058, -33.2972) (4.9075, -33.2693) knots 0 0 0 0 1 1 1 1
  spline S30 degree 3 poles (4.9075, -33.2693) (4.9091, -33.2451) (4.9103, -33.1165) (4.9103, -32.9834) knots 0 0 0 0 1 1 1 1
  spline S31 degree 3 poles (4.9103, -32.9834) (4.9103, -32.8503) (4.9091, -32.6821) (4.9075, -32.6095) knots 0 0 0 0 1 1 1 1
  line L90 (4.9075, -32.6095) -> (4.9048, -32.4775)
  line L91 (4.9048, -32.4775) -> (3.9371, -32.4775)
  line L92 (3.9371, -32.4775) -> (2.9693, -32.4775)
  line L93 (2.9693, -32.4775) -> (2.9693, -32.8954)
  spline S32 degree 3 poles (1.3409, -30.7071) (1.4251, -30.7494) (1.5389, -30.8513) (1.5938, -30.9335) knots 0 0 0 0 1 1 1 1
  spline S33 degree 3 poles (1.5938, -30.9335) (1.6926, -31.0814) (1.6937, -31.098) (1.6937, -32.55) knots 0 0 0 0 1 1 1 1
  line L94 (1.6937, -32.55) -> (1.6937, -34.0171)
  line L95 (1.6937, -34.0171) -> (1.3418, -34.0171)
  line L96 (1.3418, -34.0171) -> (0.9899, -34.0171)
  line L97 (0.9899, -34.0171) -> (0.9899, -32.6746)
  line L98 (0.9899, -32.6746) -> (0.9899, -31.3322)
  line L99 (0.9899, -31.3322) -> (0.0111, -31.344)
  line L100 (0.0111, -31.344) -> (-0.9676, -31.3558)
  line L101 (-0.9676, -31.3558) -> (-0.9792, -32.6865)
  line L102 (-0.9792, -32.6865) -> (-0.9909, -34.0171)
  line L103 (-0.9909, -34.0171) -> (-1.3438, -34.0171)
  line L104 (-1.3438, -34.0171) -> (-1.6968, -34.0171)
  line L105 (-1.6968, -34.0171) -> (-1.6841, -32.5467)
  spline S34 degree 3 poles (-1.6841, -32.5467) (-1.6719, -31.134) (-1.6678, -31.0714) (-1.5794, -30.9521) knots 0 0 0 0 1 1 1 1
  spline S35 degree 3 poles (-1.5794, -30.9521) (-1.5288, -30.8838) (-1.4219, -30.7835) (-1.3419, -30.729) knots 0 0 0 0 1 1 1 1
  spline S36 degree 3 poles (-1.3419, -30.729) (-1.2, -30.6324) (-1.1683, -30.63) (-0.0044, -30.6301) knots 0 0 0 0 1 1 1 1
  spline S37 degree 3 poles (-0.0044, -30.6301) (1.0429, -30.6302) (1.2064, -30.6395) (1.3409, -30.7071) knots 0 0 0 0 1 1 1 1
  spline S38 degree 3 poles (-2.5727, -30.729) (-2.35, -30.8806) (-2.2632, -31.0281) (-2.2348, -31.3034) knots 0 0 0 0 1 1 1 1
  line L106 (-2.2348, -31.3034) -> (-2.2089, -31.5538)
  line L107 (-2.2089, -31.5538) -> (-2.567, -31.5538)
  spline S39 degree 3 poles (-2.567, -31.5538) (-2.9196, -31.5538) (-2.9251, -31.5521) (-2.9251, -31.4438) knots 0 0 0 0 1 1 1 1
  line L108 (-2.9251, -31.4438) -> (-2.9251, -31.3339)
  line L109 (-2.9251, -31.3339) -> (-3.8928, -31.3339)
  line L110 (-3.8928, -31.3339) -> (-4.8605, -31.3339)
  line L111 (-4.8605, -31.3339) -> (-4.8605, -31.6638)
  line L112 (-4.8605, -31.6638) -> (-4.8605, -31.9937)
  line L113 (-4.8605, -31.9937) -> (-3.8268, -31.9937)
  line L114 (-3.8268, -31.9937) -> (-2.7931, -31.9937)
  line L115 (-2.7931, -31.9937) -> (-2.7931, -32.3456)
  line L116 (-2.7931, -32.3456) -> (-2.7931, -32.6975)
  line L117 (-2.7931, -32.6975) -> (-3.7608, -32.6975)
  line L118 (-3.7608, -32.6975) -> (-4.7286, -32.6975)
  line L119 (-4.7286, -32.6975) -> (-4.7286, -33.0054)
  line L120 (-4.7286, -33.0054) -> (-4.7286, -33.3133)
  line L121 (-4.7286, -33.3133) -> (-3.8268, -33.3133)
  line L122 (-3.8268, -33.3133) -> (-2.9251, -33.3133)
  line L123 (-2.9251, -33.3133) -> (-2.9251, -33.1813)
  line L124 (-2.9251, -33.1813) -> (-2.9251, -33.0494)
  line L125 (-2.9251, -33.0494) -> (-2.5732, -33.0494)
  line L126 (-2.5732, -33.0494) -> (-2.2213, -33.0494)
  line L127 (-2.2213, -33.0494) -> (-2.2215, -33.2143)
  spline S40 degree 3 poles (-2.2215, -33.2143) (-2.222, -33.4836) (-2.2987, -33.6817) (-2.4652, -33.8431) knots 0 0 0 0 1 1 1 1
  line L128 (-2.4652, -33.8431) -> (-2.6219, -33.9951)
  line L129 (-2.6219, -33.9951) -> (-3.7962, -34.0071)
  spline S41 degree 3 poles (-3.7962, -34.0071) (-4.9077, -34.0184) (-4.9782, -34.0143) (-5.1139, -33.9305) knots 0 0 0 0 1 1 1 1
  spline S42 degree 3 poles (-5.1139, -33.9305) (-5.384, -33.7637) (-5.4321, -33.6234) (-5.4323, -33.0012) knots 0 0 0 0 1 1 1 1
  spline S43 degree 3 poles (-5.4323, -33.0012) (-5.4324, -32.5846) (-5.4497, -32.4125) (-5.5019, -32.3078) knots 0 0 0 0 1 1 1 1
  spline S44 degree 3 poles (-5.5019, -32.3078) (-5.5571, -32.1972) (-5.5684, -32.0517) (-5.5569, -31.6003) knots 0 0 0 0 1 1 1 1
  spline S45 degree 3 poles (-5.5569, -31.6003) (-5.5443, -31.1087) (-5.5301, -31.0153) (-5.4513, -30.908) knots 0 0 0 0 1 1 1 1
  spline S46 degree 3 poles (-5.4513, -30.908) (-5.258, -30.6449) (-5.1753, -30.6302) (-3.8884, -30.6301) knots 0 0 0 0 1 1 1 1
  spline S47 degree 3 poles (-3.8884, -30.6301) (-2.7472, -30.63) (-2.7146, -30.6325) (-2.5728, -30.729) knots 0 0 0 0 1 1 1 1
  line L130 (-2.5728, -30.729) -> (-2.5727, -30.729)
  line L131 (12.4282, -29.8931) -> (12.3373, -30.0741)
  line L132 (11.7412, -30.8828) -> (12.0939, -30.653)
  line L133 (8.9096, -28.5153) -> (9.3429, -28.6164)
  line L134 (12.5357, -30.4255) -> (12.6248, -30.4278)
  line L135 (12.4466, -30.4233) -> (12.5357, -30.4255)
  line L136 (10.533, -29.5835) -> (10.6509, -29.1727)
  line L137 (9.8048, -28.7461) -> (9.8334, -28.7747)
  line L138 (12.0939, -30.653) -> (12.4466, -30.4233)
  line L139 (9.3429, -28.6164) -> (9.7762, -28.7175)
  line L140 (11.1403, -30.6906) -> (11.0199, -30.9104)
  line L141 (12.7501, -30.5228) -> (12.8753, -30.6179)
  line L142 (9.5797, -31.4837) -> (9.6884, -31.4848)
  line L143 (11.2216, -28.6184) -> (11.6351, -28.5196)
  line L144 (11.7993, -30.3374) -> (11.3524, -30.4198)
  line L145 (12.3905, -29.2075) -> (12.5095, -29.5396)
  line L146 (8.354, -28.866) -> (8.6318, -28.6907)
  line L147 (9.2669, -30.426) -> (9.1079, -30.389)
  line L148 (9.1079, -30.389) -> (8.9489, -30.352)
  line L149 (8.1698, -29.4484) -> (8.2047, -29.1451)
  line L150 (9.7972, -31.128) -> (9.7194, -31.0761)
  line L151 (12.6248, -30.4278) -> (12.7501, -30.5228)
  line L152 (10.7688, -28.762) -> (10.7884, -28.7396)
  line L153 (10.0925, -29.5396) -> (10.3128, -29.5616)
  line L154 (8.6318, -28.6907) -> (8.9096, -28.5153)
  line L155 (11.3524, -30.4198) -> (11.2463, -30.5552)
  line L156 (12.3373, -30.0741) -> (12.2463, -30.255)
  line L157 (9.7194, -31.0761) -> (9.6416, -31.0242)
  line L158 (11.0138, -31.413) -> (11.3775, -31.7975)
  line L159 (12.5095, -29.5396) -> (12.4689, -29.7164)
  line L160 (7.946, -30.4885) -> (8.0919, -30.3526)
  line L161 (11.1769, -33.658) -> (11.0366, -33.8263)
  line L162 (9.8846, -31.5414) -> (9.972, -31.5969)
  line L163 (11.1233, -33.3076) -> (10.8811, -33.2863)
  line L164 (8.9489, -30.352) -> (8.6661, -30.2964)
  line L165 (10.9702, -31.413) -> (10.992, -31.413)
  line L166 (10.8929, -33.5337) -> (11.0342, -33.5337)
  line L167 (10.3128, -29.5616) -> (10.533, -29.5835)
  line L168 (11.6351, -28.5196) -> (11.7058, -28.5232)
  line L169 (12.0239, -28.701) -> (12.2714, -28.8754)
  line L170 (10.8811, -33.2863) -> (10.7456, -32.9002)
  line L171 (8.178, -30.3526) -> (8.549, -30.6123)
  line L172 (11.3654, -33.3289) -> (11.1233, -33.3076)
  line L173 (10.8994, -31.1302) -> (10.3483, -31.1291)
  line L174 (8.3833, -30.2408) -> (8.2591, -29.9963)
  line L175 (10.8081, -28.7172) -> (11.2216, -28.6184)
  line L176 (11.7765, -28.5267) -> (12.0239, -28.701)
  line L177 (9.4542, -30.7251) -> (9.2669, -30.426)
  line L178 (10.8976, -33.9932) -> (10.8952, -33.7635)
  line L179 (8.2591, -29.9963) -> (8.1349, -29.7517)
  line L180 (8.2047, -29.1451) -> (8.2794, -29.0056)
  line L181 (8.549, -30.6123) -> (8.92, -30.8721)
  line L182 (10.7884, -28.7396) -> (10.8081, -28.7172)
  line L183 (8.1349, -30.3526) -> (8.178, -30.3526)
  line L184 (12.2463, -30.255) -> (11.7993, -30.3374)
  line L185 (9.7762, -28.7175) -> (9.8048, -28.7461)
  line L186 (11.0366, -33.8263) -> (10.8976, -33.9932)
  line L187 (11.1756, -33.5966) -> (11.1769, -33.658)
  line L188 (8.1349, -29.7517) -> (8.1698, -29.4484)
  line L189 (8.6661, -30.2964) -> (8.3833, -30.2408)
  line L190 (12.4689, -29.7164) -> (12.4282, -29.8931)
  line L191 (10.6101, -32.5141) -> (10.6101, -32.0456)
  line L192 (11.2463, -30.5552) -> (11.1403, -30.6906)
  line L193 (11.7058, -28.5232) -> (11.7765, -28.5267)
  line L194 (8.0919, -30.3526) -> (8.1349, -30.3526)
  line L195 (12.8753, -30.6179) -> (12.9185, -31.1776)
  line L196 (9.6301, -33.3923) -> (9.4361, -33.3923)
  line L197 (10.6101, -32.0456) -> (10.6101, -31.5771)
  line L198 (7.7498, -31.1608) -> (7.8001, -30.6244)
  line L199 (12.3719, -32.1906) -> (12.0859, -31.9238)
  line L200 (9.8242, -33.3923) -> (9.6301, -33.3923)
  line L201 (9.6416, -31.0242) -> (9.4542, -30.7251)
  line L202 (7.9663, -32.1552) -> (7.8329, -31.9262)
  line L203 (9.7651, -33.9579) -> (9.6453, -33.7751)
  line L204 (9.5256, -33.5924) -> (9.626, -33.5288)
  line L205 (10.0864, -32.438) -> (10.0073, -32.8309)
  line L206 (8.9829, -32.9248) -> (8.9579, -32.646)
  line L207 (9.2095, -33.1586) -> (8.9829, -32.9248)
  line L208 (9.0782, -32.0845) -> (9.3289, -31.7841)
  line L209 (11.7705, -31.2699) -> (11.7412, -30.8828)
  line L210 (11.3775, -31.7975) -> (11.7412, -32.1821)
  line L211 (8.2501, -32.1968) -> (8.1082, -32.176)
  line L212 (8.2066, -32.8551) -> (8.1409, -32.7879)
  line L213 (8.0929, -32.332) -> (8.2066, -32.332)
  line L214 (11.0199, -30.9104) -> (10.8994, -31.1302)
  line L215 (9.626, -33.5288) -> (9.7265, -33.4652)
  line L216 (8.92, -30.8721) -> (8.9055, -31.2746)
  line L217 (8.1409, -32.7879) -> (8.0752, -32.7208)
  line L218 (7.9792, -32.332) -> (8.0929, -32.332)
  line L219 (8.0752, -32.7208) -> (8.0272, -32.5264)
  line L220 (8.1082, -32.176) -> (7.9663, -32.1552)
  line L221 (9.972, -31.5969) -> (10.0292, -32.0174)
  line L222 (9.6453, -33.7751) -> (9.5256, -33.5924)
  line L223 (8.0272, -32.5264) -> (7.9792, -32.332)
  line L224 (12.9616, -31.7373) -> (12.8444, -31.9639)
  line L225 (8.5705, -31.937) -> (8.2501, -32.1968)
  line L226 (12.5496, -32.1906) -> (12.3719, -32.1906)
  line L227 (10.8952, -33.7635) -> (10.8929, -33.5337)
  line L228 (10.6509, -29.1727) -> (10.7688, -28.762)
  line L229 (12.4498, -32.3299) -> (12.4498, -32.5914)
  line L230 (12.9185, -31.1776) -> (12.9616, -31.7373)
  line L231 (11.0342, -33.5337) -> (11.1756, -33.5337)
  line L232 (9.8334, -28.7747) -> (9.963, -29.1572)
  line L233 (8.9055, -31.2746) -> (8.891, -31.6771)
  line L234 (8.9329, -32.3673) -> (9.0055, -32.2259)
  line L235 (12.4498, -32.5914) -> (12.4498, -32.853)
  line L236 (12.5812, -32.7187) -> (12.6292, -32.5243)
  line L237 (7.8329, -31.9262) -> (7.6996, -31.6971)
  line L238 (9.0055, -32.2259) -> (9.0782, -32.0845)
  line L239 (9.963, -29.1572) -> (10.0925, -29.5396)
  line L240 (10.3483, -31.1291) -> (9.7972, -31.128)
  line L241 (8.2066, -32.5935) -> (8.2066, -32.8551)
  line L242 (9.8325, -33.463) -> (9.8325, -33.7105)
  line L243 (8.891, -31.6771) -> (8.5705, -31.937)
  line L244 (10.7902, -31.495) -> (10.9702, -31.413)
  line L245 (11.7412, -32.8362) -> (11.5533, -33.0825)
  line L246 (11.5533, -33.0825) -> (11.3654, -33.3289)
  line L247 (12.8444, -31.9639) -> (12.7272, -32.1906)
  line L248 (12.6292, -32.5243) -> (12.6772, -32.3299)
  line L249 (10.992, -31.413) -> (11.0138, -31.413)
  line L250 (9.7988, -33.9579) -> (9.7651, -33.9579)
  line L251 (9.4361, -33.3923) -> (9.2095, -33.1586)
  line L252 (8.2794, -29.0056) -> (8.354, -28.866)
  line L253 (9.7795, -33.4641) -> (9.8325, -33.463)
  line L254 (7.6996, -31.6971) -> (7.7498, -31.1608)
  line L255 (12.6772, -32.3299) -> (12.5635, -32.3299)
  line L256 (12.2714, -28.8754) -> (12.3905, -29.2075)
  line L257 (11.7412, -32.5092) -> (11.7412, -32.8362)
  line L258 (12.7272, -32.1906) -> (12.5496, -32.1906)
  line L259 (12.0859, -31.9238) -> (11.7999, -31.657)
  line L260 (9.7972, -31.4858) -> (9.8846, -31.5414)
  line L261 (10.7456, -32.9002) -> (10.6101, -32.5141)
  line L262 (7.8001, -30.6244) -> (7.946, -30.4885)
  line L263 (9.8762, -33.3081) -> (9.8242, -33.3923)
  line L264 (9.8325, -33.9579) -> (9.7988, -33.9579)
  line L265 (10.0292, -32.0174) -> (10.0864, -32.438)
  line L266 (9.6884, -31.4848) -> (9.7972, -31.4858)
  line L267 (11.1756, -33.5337) -> (11.1756, -33.5966)
  line L268 (9.3289, -31.7841) -> (9.5797, -31.4837)
  line L269 (11.7412, -32.1821) -> (11.7412, -32.5092)
  line L270 (12.4498, -32.853) -> (12.5155, -32.7858)
  line L271 (8.9579, -32.646) -> (8.9329, -32.3673)
  line L272 (12.5635, -32.3299) -> (12.4498, -32.3299)
  line L273 (9.7265, -33.4652) -> (9.7795, -33.4641)
  line L274 (8.2066, -32.332) -> (8.2066, -32.5935)
  line L275 (9.8325, -33.7105) -> (9.8325, -33.9579)
  line L276 (10.6101, -31.5771) -> (10.7902, -31.495)
  line L277 (11.7999, -31.657) -> (11.7705, -31.2699)
  line L278 (12.5155, -32.7858) -> (12.5812, -32.7187)
  line L279 (10.0073, -32.8309) -> (9.9283, -33.2239)
  line L280 (9.9283, -33.2239) -> (9.8762, -33.3081)
  constraint coincident L187.start L267.end
emboss "Gravure en relief3" depth 0.3 profiles "Esquisse9" section 1 onto face at (9.9503, -32.5, -100.9957) on bodies 7 bodies 7
pattern_circular "Réseau C1" count 3 over 360 about axis through (0, -35, -100) along (0, 1, 0) of "Gravure en relief3"
